Autodesk Inventor part; units mm, degrees
(part 2 of 3)
  spline S168 degree 2 poles (47.2484, 57.1416) (47.3031, 57.1416) (47.4113, 57.1684) (47.4635, 57.189) knots 0 0 0 1 2 2 2
  spline S169 degree 2 poles (47.4635, 57.189) (47.5122, 57.2097) (47.5839, 57.2534) (47.6118, 57.2729) knots 0 0 0 1 2 2 2
  line L293 (47.6118, 57.2729) -> (47.624, 57.2729)
  line L294 (47.624, 57.2729) -> (47.624, 57.0602)
  spline S170 degree 2 poles (47.624, 57.0602) (47.5583, 57.0249) (47.3335, 56.9678) (47.2326, 56.9678) knots 0 0 0 1 2 2 2
  spline S171 degree 2 poles (47.2326, 56.9678) (47.1305, 56.9678) (46.9785, 57.0091) (46.9165, 57.0529) knots 0 0 0 1 2 2 2
  spline S172 degree 2 poles (46.9165, 57.0529) (46.8509, 57.1003) (46.7828, 57.2376) (46.7828, 57.33) knots 0 0 0 1 2 2 2
  spline S173 degree 2 poles (46.7828, 57.33) (46.7828, 57.454) (46.9457, 57.6412) (47.06, 57.6655) knots 0 0 0 1 2 2 2
  line L295 (47.06, 57.6655) -> (47.06, 57.6801)
  spline S174 degree 2 poles (47.06, 57.6801) (47.0126, 57.6898) (46.9044, 57.7336) (46.8582, 57.7774) knots 0 0 0 1 2 2 2
  spline S175 degree 2 poles (46.8582, 57.7774) (46.812, 57.8199) (46.7536, 57.956) (46.7536, 58.0545) knots 0 0 0 1 2 2 2
  spline S176 degree 2 poles (46.7536, 58.0545) (46.7536, 58.1554) (46.8229, 58.3268) (46.8861, 58.3924) knots 0 0 0 1 2 2 2
  spline S177 degree 2 poles (46.8861, 58.3924) (46.9518, 58.4605) (47.1378, 58.531) (47.2557, 58.531) knots 0 0 0 1 2 2 2
  spline S178 degree 2 poles (47.2557, 58.531) (47.3687, 58.531) (47.59, 58.4763) (47.6653, 58.4386) knots 0 0 0 1 2 2 2
  line L296 (47.6653, 58.4386) -> (47.6653, 58.2259)
  line L297 (47.6653, 58.2259) -> (47.6507, 58.2259)
  spline S179 degree 2 poles (47.6507, 58.2259) (47.5875, 58.2721) (47.3736, 58.3572) (47.2678, 58.3572) knots 0 0 0 1 2 2 2
  spline S180 degree 2 poles (47.2678, 58.3572) (47.2058, 58.3572) (47.0818, 58.3183) (47.0405, 58.2733) knots 0 0 0 1 2 2 2
  spline S181 degree 2 poles (47.0405, 58.2733) (47.0004, 58.2283) (46.9579, 58.1214) (46.9579, 58.0399) knots 0 0 0 1 2 2 2
  spline S182 degree 2 poles (46.9579, 58.0399) (46.9579, 57.9585) (47.0053, 57.8527) (47.0478, 57.8223) knots 0 0 0 1 2 2 2
  spline S183 degree 2 poles (47.0478, 57.8223) (47.0904, 57.7919) (47.2058, 57.7688) (47.2739, 57.7688) knots 0 0 0 1 2 2 2
  line L298 (47.2739, 57.7688) -> (47.359, 57.7688)
  line L299 (47.359, 57.7688) -> (47.359, 57.6023)
  line L300 (47.359, 57.6023) -> (47.2921, 57.6023)
  spline S184 degree 2 poles (47.2921, 57.6023) (47.1572, 57.6023) (46.987, 57.4735) (46.987, 57.3507) knots 0 0 0 1 2 2 2
  spline S185 degree 2 poles (46.987, 57.3507) (46.987, 57.2936) (47.0308, 57.2121) (47.066, 57.1878) knots 0 0 0 1 2 2 2
  spline S186 degree 2 poles (47.066, 57.1878) (47.1037, 57.1623) (47.1961, 57.1416) (47.2484, 57.1416) knots 0 0 0 1 2 2 2
  line L301 (49.0097, 60.9994) -> (48.5041, 59.4994)
  line L302 (48.5041, 59.4994) -> (48.2585, 59.4994)
  line L303 (48.2585, 59.4994) -> (47.7528, 60.9994)
  line L304 (47.7528, 60.9994) -> (47.9631, 60.9994)
  line L305 (47.9631, 60.9994) -> (48.0993, 60.58)
  line L306 (48.0993, 60.58) -> (48.6718, 60.58)
  line L307 (48.6718, 60.58) -> (48.8079, 60.9994)
  line L308 (48.8079, 60.9994) -> (49.0097, 60.9994)
  line L309 (48.154, 60.4098) -> (48.3861, 59.7036)
  line L310 (48.3861, 59.7036) -> (48.6171, 60.4098)
  line L311 (48.6171, 60.4098) -> (48.154, 60.4098)
  line L312 (46.688, 60.484) -> (46.8667, 60.484)
  line L313 (46.8667, 60.484) -> (46.8667, 60.9994)
  line L314 (46.8667, 60.9994) -> (47.06, 60.9994)
  line L315 (47.06, 60.9994) -> (47.06, 60.484)
  line L316 (47.06, 60.484) -> (47.7224, 60.484)
  line L317 (47.7224, 60.484) -> (47.7224, 60.2725)
  line L318 (47.7224, 60.2725) -> (47.0515, 59.4994)
  line L319 (47.0515, 59.4994) -> (46.8667, 59.4994)
  line L320 (46.8667, 59.4994) -> (46.8667, 60.3223)
  line L321 (46.8667, 60.3223) -> (46.688, 60.3223)
  line L322 (46.688, 60.3223) -> (46.688, 60.484)
  line L323 (47.06, 60.3223) -> (47.06, 59.7364)
  line L324 (47.06, 59.7364) -> (47.5644, 60.3223)
  line L325 (47.5644, 60.3223) -> (47.06, 60.3223)
  line L326 (49.0097, 63.4994) -> (48.5041, 61.9994)
  line L327 (48.5041, 61.9994) -> (48.2585, 61.9994)
  line L328 (48.2585, 61.9994) -> (47.7528, 63.4994)
  line L329 (47.7528, 63.4994) -> (47.9631, 63.4994)
  line L330 (47.9631, 63.4994) -> (48.0993, 63.08)
  line L331 (48.0993, 63.08) -> (48.6718, 63.08)
  line L332 (48.6718, 63.08) -> (48.8079, 63.4994)
  line L333 (48.8079, 63.4994) -> (49.0097, 63.4994)
  line L334 (48.154, 62.9098) -> (48.3861, 62.2036)
  line L335 (48.3861, 62.2036) -> (48.6171, 62.9098)
  line L336 (48.6171, 62.9098) -> (48.154, 62.9098)
  spline S187 degree 2 poles (46.7439, 63.0229) (46.7439, 63.1311) (46.8132, 63.3158) (46.8764, 63.3839) knots 0 0 0 1 2 2 2
  spline S188 degree 2 poles (46.8764, 63.3839) (46.9396, 63.452) (47.128, 63.531) (47.2447, 63.531) knots 0 0 0 1 2 2 2
  spline S189 degree 2 poles (47.2447, 63.531) (47.3517, 63.531) (47.5608, 63.4836) (47.6374, 63.4459) knots 0 0 0 1 2 2 2
  line L337 (47.6374, 63.4459) -> (47.6374, 63.2332)
  line L338 (47.6374, 63.2332) -> (47.6228, 63.2332)
  spline S190 degree 2 poles (47.6228, 63.2332) (47.5997, 63.2502) (47.5134, 63.294) (47.4611, 63.3134) knots 0 0 0 1 2 2 2
  spline S191 degree 2 poles (47.4611, 63.3134) (47.4015, 63.3341) (47.3031, 63.3572) (47.2411, 63.3572) knots 0 0 0 1 2 2 2
  spline S192 degree 2 poles (47.2411, 63.3572) (47.1803, 63.3572) (47.066, 63.3134) (47.0247, 63.266) knots 0 0 0 1 2 2 2
  spline S193 degree 2 poles (47.0247, 63.266) (46.987, 63.221) (46.9481, 63.1019) (46.9481, 63.0217) knots 0 0 0 1 2 2 2
  spline S194 degree 2 poles (46.9481, 63.0217) (46.9481, 62.9415) (46.9919, 62.8393) (47.0332, 62.8053) knots 0 0 0 1 2 2 2
  spline S195 degree 2 poles (47.0332, 62.8053) (47.0758, 62.7676) (47.2022, 62.736) (47.2788, 62.736) knots 0 0 0 1 2 2 2
  spline S196 degree 2 poles (47.2788, 62.736) (47.3614, 62.736) (47.5255, 62.7615) (47.5754, 62.7725) knots 0 0 0 1 2 2 2
  line L339 (47.5754, 62.7725) -> (47.5754, 61.9994)
  line L340 (47.5754, 61.9994) -> (46.7524, 61.9994)
  line L341 (46.7524, 61.9994) -> (46.7524, 62.1756)
  line L342 (46.7524, 62.1756) -> (47.3821, 62.1756)
  line L343 (47.3821, 62.1756) -> (47.3821, 62.5756)
  spline S197 degree 2 poles (47.3821, 62.5756) (47.3456, 62.5707) (47.2751, 62.5671) (47.2459, 62.5671) knots 0 0 0 1 2 2 2
  spline S198 degree 2 poles (47.2459, 62.5671) (47.1305, 62.5671) (46.9712, 62.6047) (46.8983, 62.6607) knots 0 0 0 1 2 2 2
  spline S199 degree 2 poles (46.8983, 62.6607) (46.8241, 62.7166) (46.7439, 62.8868) (46.7439, 63.0229) knots 0 0 0 1 2 2 2
  line L344 (8.7601, 25.608) -> (8.2545, 24.108)
  line L345 (8.2545, 24.108) -> (8.0089, 24.108)
  line L346 (8.0089, 24.108) -> (7.5032, 25.608)
  line L347 (7.5032, 25.608) -> (7.7135, 25.608)
  line L348 (7.7135, 25.608) -> (7.8497, 25.1886)
  line L349 (7.8497, 25.1886) -> (8.4222, 25.1886)
  line L350 (8.4222, 25.1886) -> (8.5583, 25.608)
  line L351 (8.5583, 25.608) -> (8.7601, 25.608)
  line L352 (7.9044, 25.0184) -> (8.1365, 24.3122)
  line L353 (8.1365, 24.3122) -> (8.3675, 25.0184)
  line L354 (8.3675, 25.0184) -> (7.9044, 25.0184)
  line L355 (6.2002, 25.608) -> (6.4591, 25.608)
  line L356 (6.4591, 25.608) -> (6.9331, 25.0111)
  line L357 (6.9331, 25.0111) -> (7.1617, 25.0111)
  line L358 (7.1617, 25.0111) -> (7.1617, 25.608)
  line L359 (7.1617, 25.608) -> (7.361, 25.608)
  line L360 (7.361, 25.608) -> (7.361, 24.108)
  line L361 (7.361, 24.108) -> (6.9745, 24.108)
  spline S200 degree 2 poles (6.9745, 24.108) (6.8456, 24.108) (6.6718, 24.1359) (6.5928, 24.187) knots 0 0 0 1 2 2 2
  spline S201 degree 2 poles (6.5928, 24.187) (6.5138, 24.238) (6.4226, 24.3973) (6.4226, 24.5152) knots 0 0 0 1 2 2 2
  spline S202 degree 2 poles (6.4226, 24.5152) (6.4226, 24.6793) (6.5904, 24.9017) (6.7338, 24.9552) knots 0 0 0 1 2 2 2
  line L362 (6.7338, 24.9552) -> (6.2002, 25.608)
  spline S203 degree 2 poles (6.6305, 24.531) (6.6305, 24.4654) (6.6767, 24.3645) (6.7253, 24.3316) knots 0 0 0 1 2 2 2
  spline S204 degree 2 poles (6.7253, 24.3316) (6.7678, 24.3037) (6.8809, 24.2806) (6.9635, 24.2806) knots 0 0 0 1 2 2 2
  line L363 (6.9635, 24.2806) -> (7.1617, 24.2806)
  line L364 (7.1617, 24.2806) -> (7.1617, 24.8446)
  line L365 (7.1617, 24.8446) -> (6.9866, 24.8446)
  spline S205 degree 2 poles (6.9866, 24.8446) (6.9003, 24.8446) (6.763, 24.8142) (6.7156, 24.7668) knots 0 0 0 1 2 2 2
  spline S206 degree 2 poles (6.7156, 24.7668) (6.6718, 24.7255) (6.6305, 24.6088) (6.6305, 24.531) knots 0 0 0 1 2 2 2
  line L366 (6.081, 25.608) -> (6.081, 24.108)
  line L367 (6.081, 24.108) -> (5.1426, 24.108)
  line L368 (5.1426, 24.108) -> (5.1426, 24.2855)
  line L369 (5.1426, 24.2855) -> (5.8817, 24.2855)
  line L370 (5.8817, 24.2855) -> (5.8817, 24.6963)
  line L371 (5.8817, 24.6963) -> (5.1925, 24.6963)
  line L372 (5.1925, 24.6963) -> (5.1925, 24.8738)
  line L373 (5.1925, 24.8738) -> (5.8817, 24.8738)
  line L374 (5.8817, 24.8738) -> (5.8817, 25.4305)
  line L375 (5.8817, 25.4305) -> (5.1426, 25.4305)
  line L376 (5.1426, 25.4305) -> (5.1426, 25.608)
  line L377 (5.1426, 25.608) -> (6.081, 25.608)
  line L378 (4.0267, 24.2855) -> (4.7245, 24.2855)
  line L379 (4.7245, 24.2855) -> (4.7245, 24.7085)
  line L380 (4.7245, 24.7085) -> (4.0559, 24.7085)
  line L381 (4.0559, 24.7085) -> (4.0559, 24.8859)
  line L382 (4.0559, 24.8859) -> (4.7245, 24.8859)
  line L383 (4.7245, 24.8859) -> (4.7245, 25.608)
  line L384 (4.7245, 25.608) -> (4.9238, 25.608)
  line L385 (4.9238, 25.608) -> (4.9238, 24.108)
  line L386 (4.9238, 24.108) -> (4.0267, 24.108)
  line L387 (4.0267, 24.108) -> (4.0267, 24.2855)
  spline S207 degree 2 poles (7.3732, 28.1372) (7.5324, 28.1372) (7.7962, 28.0399) (7.891, 27.9415) knots 0 0 0 1 2 2 2
  spline S208 degree 2 poles (7.891, 27.9415) (7.9858, 27.8418) (8.0867, 27.5476) (8.0867, 27.3568) knots 0 0 0 1 2 2 2
  spline S209 degree 2 poles (8.0867, 27.3568) (8.0867, 27.1756) (7.9846, 26.8888) (7.8898, 26.7867) knots 0 0 0 1 2 2 2
  spline S210 degree 2 poles (7.8898, 26.7867) (7.7986, 26.6882) (7.5312, 26.5812) (7.372, 26.5812) knots 0 0 0 1 2 2 2
  spline S211 degree 2 poles (7.372, 26.5812) (7.2954, 26.5812) (7.1568, 26.6031) (7.0936, 26.6226) knots 0 0 0 1 2 2 2
  spline S212 degree 2 poles (7.0936, 26.6226) (7.0425, 26.6372) (6.9186, 26.6906) (6.8809, 26.7101) knots 0 0 0 1 2 2 2
  line L388 (6.8809, 26.7101) -> (6.8809, 26.9508)
  line L389 (6.8809, 26.9508) -> (6.8979, 26.9508)
  spline S213 degree 2 poles (6.8979, 26.9508) (6.9356, 26.9179) (7.0146, 26.8584) (7.0875, 26.8244) knots 0 0 0 1 2 2 2
  spline S214 degree 2 poles (7.0875, 26.8244) (7.1483, 26.794) (7.3051, 26.7538) (7.3951, 26.7538) knots 0 0 0 1 2 2 2
  spline S215 degree 2 poles (7.3951, 26.7538) (7.6114, 26.7538) (7.8788, 27.0796) (7.8788, 27.3507) knots 0 0 0 1 2 2 2
  spline S216 degree 2 poles (7.8788, 27.3507) (7.8788, 27.5014) (7.8083, 27.7275) (7.7415, 27.8053) knots 0 0 0 1 2 2 2
  spline S217 degree 2 poles (7.7415, 27.8053) (7.6771, 27.8831) (7.4947, 27.9645) (7.3805, 27.9645) knots 0 0 0 1 2 2 2
  spline S218 degree 2 poles (7.3805, 27.9645) (7.2966, 27.9645) (7.1288, 27.9402) (7.0717, 27.9159) knots 0 0 0 1 2 2 2
  line L390 (7.0717, 27.9159) -> (7.0717, 27.5282)
  line L391 (7.0717, 27.5282) -> (7.4194, 27.5282)
  line L392 (7.4194, 27.5282) -> (7.4194, 27.3531)
  line L393 (7.4194, 27.3531) -> (6.8748, 27.3531)
  line L394 (6.8748, 27.3531) -> (6.8748, 28.0083)
  spline S219 degree 2 poles (6.8748, 28.0083) (6.9125, 28.0253) (7.0413, 28.0776) (7.096, 28.0934) knots 0 0 0 1 2 2 2
  spline S220 degree 2 poles (7.096, 28.0934) (7.1702, 28.1153) (7.2893, 28.1372) (7.3732, 28.1372) knots 0 0 0 1 2 2 2
  line L395 (5.5511, 28.108) -> (5.7747, 28.108)
  line L396 (5.7747, 28.108) -> (6.4384, 26.8146)
  line L397 (6.4384, 26.8146) -> (6.4384, 28.108)
  line L398 (6.4384, 28.108) -> (6.6244, 28.108)
  line L399 (6.6244, 28.108) -> (6.6244, 26.608)
  line L400 (6.6244, 26.608) -> (6.3412, 26.608)
  line L401 (6.3412, 26.608) -> (5.737, 27.7956)
  line L402 (5.737, 27.7956) -> (5.737, 26.608)
  line L403 (5.737, 26.608) -> (5.5511, 26.608)
  line L404 (5.5511, 26.608) -> (5.5511, 28.108)
  spline S221 degree 2 poles (4.0644, 27.3592) (4.0644, 27.5646) (4.231, 27.8953) (4.3707, 27.9876) knots 0 0 0 1 2 2 2
  spline S222 degree 2 poles (4.3707, 27.9876) (4.485, 28.0594) (4.7196, 28.108) (4.9019, 28.108) knots 0 0 0 1 2 2 2
  line L405 (4.9019, 28.108) -> (5.2472, 28.108)
  line L406 (5.2472, 28.108) -> (5.2472, 26.608)
  line L407 (5.2472, 26.608) -> (4.9056, 26.608)
  spline S223 degree 2 poles (4.9056, 26.608) (4.6941, 26.608) (4.4534, 26.6712) (4.3683, 26.7271) knots 0 0 0 1 2 2 2
  spline S224 degree 2 poles (4.3683, 26.7271) (4.2237, 26.8231) (4.0644, 27.1404) (4.0644, 27.3592) knots 0 0 0 1 2 2 2
  spline S225 degree 2 poles (4.2723, 27.3568) (4.2723, 27.1842) (4.3865, 26.9398) (4.4996, 26.8705) knots 0 0 0 1 2 2 2
  spline S226 degree 2 poles (4.4996, 26.8705) (4.5798, 26.8231) (4.7609, 26.7806) (4.8959, 26.7806) knots 0 0 0 1 2 2 2
  line L408 (4.8959, 26.7806) -> (5.0478, 26.7806)
  line L409 (5.0478, 26.7806) -> (5.0478, 27.9354)
  line L410 (5.0478, 27.9354) -> (4.8959, 27.9354)
  spline S227 degree 2 poles (4.8959, 27.9354) (4.7634, 27.9354) (4.5628, 27.8928) (4.4814, 27.8357) knots 0 0 0 1 2 2 2
  spline S228 degree 2 poles (4.4814, 27.8357) (4.3768, 27.7652) (4.2723, 27.5318) (4.2723, 27.3568) knots 0 0 0 1 2 2 2
  line L411 (5.2921, 30.608) -> (6.0239, 30.608)
  line L412 (6.0239, 30.608) -> (6.0239, 30.4548)
  line L413 (6.0239, 30.4548) -> (5.7516, 30.4548)
  line L414 (5.7516, 30.4548) -> (5.7516, 29.4496)
  line L415 (5.7516, 29.4496) -> (6.0239, 29.4496)
  line L416 (6.0239, 29.4496) -> (6.0239, 29.3122)
  spline S229 degree 2 poles (6.0239, 29.3122) (5.8695, 29.3122) (5.7237, 29.2247) (5.7139, 29.1031) knots 0 0 0 1 2 2 2
  line L417 (5.7139, 29.1031) -> (5.5583, 29.1031)
  line L418 (5.5583, 29.1031) -> (5.5583, 30.4548)
  line L419 (5.5583, 30.4548) -> (5.2921, 30.4548)
  line L420 (5.2921, 30.4548) -> (5.2921, 30.608)
  spline S230 degree 2 poles (4.6114, 29.2502) (4.6661, 29.2502) (4.7743, 29.2769) (4.8266, 29.2976) knots 0 0 0 1 2 2 2
  spline S231 degree 2 poles (4.8266, 29.2976) (4.8752, 29.3183) (4.9469, 29.362) (4.9749, 29.3815) knots 0 0 0 1 2 2 2
  line L421 (4.9749, 29.3815) -> (4.987, 29.3815)
  line L422 (4.987, 29.3815) -> (4.987, 29.1688)
  spline S232 degree 2 poles (4.987, 29.1688) (4.9214, 29.1335) (4.6965, 29.0764) (4.5956, 29.0764) knots 0 0 0 1 2 2 2
  spline S233 degree 2 poles (4.5956, 29.0764) (4.4935, 29.0764) (4.3416, 29.1177) (4.2796, 29.1615) knots 0 0 0 1 2 2 2
  spline S234 degree 2 poles (4.2796, 29.1615) (4.2139, 29.2089) (4.1459, 29.3462) (4.1459, 29.4386) knots 0 0 0 1 2 2 2
  spline S235 degree 2 poles (4.1459, 29.4386) (4.1459, 29.5626) (4.3088, 29.7498) (4.423, 29.7741) knots 0 0 0 1 2 2 2
  line L423 (4.423, 29.7741) -> (4.423, 29.7887)
  spline S236 degree 2 poles (4.423, 29.7887) (4.3756, 29.7984) (4.2674, 29.8422) (4.2212, 29.8859) knots 0 0 0 1 2 2 2
  spline S237 degree 2 poles (4.2212, 29.8859) (4.175, 29.9285) (4.1167, 30.0646) (4.1167, 30.1631) knots 0 0 0 1 2 2 2
  spline S238 degree 2 poles (4.1167, 30.1631) (4.1167, 30.264) (4.186, 30.4354) (4.2492, 30.501) knots 0 0 0 1 2 2 2
  spline S239 degree 2 poles (4.2492, 30.501) (4.3148, 30.5691) (4.5008, 30.6396) (4.6187, 30.6396) knots 0 0 0 1 2 2 2
  spline S240 degree 2 poles (4.6187, 30.6396) (4.7318, 30.6396) (4.953, 30.5849) (5.0284, 30.5472) knots 0 0 0 1 2 2 2
  line L424 (5.0284, 30.5472) -> (5.0284, 30.3345)
  line L425 (5.0284, 30.3345) -> (5.0138, 30.3345)
  spline S241 degree 2 poles (5.0138, 30.3345) (4.9506, 30.3807) (4.7366, 30.4658) (4.6309, 30.4658) knots 0 0 0 1 2 2 2
  spline S242 degree 2 poles (4.6309, 30.4658) (4.5689, 30.4658) (4.4449, 30.4269) (4.4036, 30.3819) knots 0 0 0 1 2 2 2
  spline S243 degree 2 poles (4.4036, 30.3819) (4.3635, 30.3369) (4.3209, 30.2299) (4.3209, 30.1485) knots 0 0 0 1 2 2 2
  spline S244 degree 2 poles (4.3209, 30.1485) (4.3209, 30.0671) (4.3683, 29.9613) (4.4109, 29.9309) knots 0 0 0 1 2 2 2
  spline S245 degree 2 poles (4.4109, 29.9309) (4.4534, 29.9005) (4.5689, 29.8774) (4.637, 29.8774) knots 0 0 0 1 2 2 2
  line L426 (4.637, 29.8774) -> (4.722, 29.8774)
  line L427 (4.722, 29.8774) -> (4.722, 29.7109)
  line L428 (4.722, 29.7109) -> (4.6552, 29.7109)
  spline S246 degree 2 poles (4.6552, 29.7109) (4.5203, 29.7109) (4.3501, 29.5821) (4.3501, 29.4593) knots 0 0 0 1 2 2 2
  spline S247 degree 2 poles (4.3501, 29.4593) (4.3501, 29.4021) (4.3938, 29.3207) (4.4291, 29.2964) knots 0 0 0 1 2 2 2
  spline S248 degree 2 poles (4.4291, 29.2964) (4.4668, 29.2709) (4.5592, 29.2502) (4.6114, 29.2502) knots 0 0 0 1 2 2 2
  line L429 (5.2921, 33.108) -> (6.0239, 33.108)
  line L430 (6.0239, 33.108) -> (6.0239, 32.9548)
  line L431 (6.0239, 32.9548) -> (5.7516, 32.9548)
  line L432 (5.7516, 32.9548) -> (5.7516, 31.9496)
  line L433 (5.7516, 31.9496) -> (6.0239, 31.9496)
  line L434 (6.0239, 31.9496) -> (6.0239, 31.8122)
  spline S249 degree 2 poles (6.0239, 31.8122) (5.8695, 31.8122) (5.7237, 31.7247) (5.7139, 31.6031) knots 0 0 0 1 2 2 2
  line L435 (5.7139, 31.6031) -> (5.5583, 31.6031)
  line L436 (5.5583, 31.6031) -> (5.5583, 32.9548)
  line L437 (5.5583, 32.9548) -> (5.2921, 32.9548)
  line L438 (5.2921, 32.9548) -> (5.2921, 33.108)
  line L439 (4.0912, 33.108) -> (5.0162, 33.108)
  line L440 (5.0162, 33.108) -> (5.0162, 32.8953)
  spline S250 degree 2 poles (5.0162, 32.8953) (4.9165, 32.8017) (4.7391, 32.6278) (4.654, 32.5342) knots 0 0 0 1 2 2 2
  spline S251 degree 2 poles (4.654, 32.5342) (4.4826, 32.3458) (4.3574, 32.1197) (4.3574, 31.9994) knots 0 0 0 1 2 2 2
  spline S252 degree 2 poles (4.3574, 31.9994) (4.3574, 31.9362) (4.3963, 31.8414) (4.4315, 31.811) knots 0 0 0 1 2 2 2
  spline S253 degree 2 poles (4.4315, 31.811) (4.4668, 31.7806) (4.5592, 31.7502) (4.6151, 31.7502) knots 0 0 0 1 2 2 2
  spline S254 degree 2 poles (4.6151, 31.7502) (4.6686, 31.7502) (4.778, 31.7769) (4.8278, 31.7976) knots 0 0 0 1 2 2 2
  spline S255 degree 2 poles (4.8278, 31.7976) (4.8703, 31.8146) (4.9494, 31.8632) (4.9737, 31.8803) knots 0 0 0 1 2 2 2
  line L441 (4.9737, 31.8803) -> (4.9846, 31.8803)
  line L442 (4.9846, 31.8803) -> (4.9846, 31.6663)
  spline S256 degree 2 poles (4.9846, 31.6663) (4.9226, 31.6359) (4.7002, 31.5764) (4.6005, 31.5764) knots 0 0 0 1 2 2 2
  spline S257 degree 2 poles (4.6005, 31.5764) (4.3902, 31.5764) (4.1532, 31.7988) (4.1532, 31.9885) knots 0 0 0 1 2 2 2
  spline S258 degree 2 poles (4.1532, 31.9885) (4.1532, 32.0772) (4.1945, 32.2255) (4.231, 32.2887) knots 0 0 0 1 2 2 2
  spline S259 degree 2 poles (4.231, 32.2887) (4.2674, 32.3543) (4.3732, 32.4832) (4.4315, 32.5452) knots 0 0 0 1 2 2 2
  spline S260 degree 2 poles (4.4315, 32.5452) (4.5263, 32.6485) (4.7585, 32.8697) (4.8278, 32.9342) knots 0 0 0 1 2 2 2
  line L443 (4.8278, 32.9342) -> (4.0912, 32.9342)
  line L444 (4.0912, 32.9342) -> (4.0912, 33.108)
  spline S261 degree 2 poles (6.3861, 34.6756) (6.3886, 34.7778) (6.4263, 34.9686) (6.4676, 35.044) knots 0 0 0 1 2 2 2
  spline S262 degree 2 poles (6.4676, 35.044) (6.5089, 35.1169) (6.6317, 35.2093) (6.7301, 35.2093) knots 0 0 0 1 2 2 2
  spline S263 degree 2 poles (6.7301, 35.2093) (6.7885, 35.2093) (6.8797, 35.1777) (6.9149, 35.1534) knots 0 0 0 1 2 2 2
  spline S264 degree 2 poles (6.9149, 35.1534) (6.9502, 35.1278) (7.0146, 35.0573) (7.0401, 35.0269) knots 0 0 0 1 2 2 2
  spline S265 degree 2 poles (7.0401, 35.0269) (7.0669, 34.9941) (7.1191, 34.9248) (7.1447, 34.8993) knots 0 0 0 1 2 2 2
  spline S266 degree 2 poles (7.1447, 34.8993) (7.1726, 34.8714) (7.231, 34.8373) (7.2674, 34.8373) knots 0 0 0 1 2 2 2
  spline S267 degree 2 poles (7.2674, 34.8373) (7.3185, 34.8373) (7.3853, 34.8908) (7.4072, 34.9431) knots 0 0 0 1 2 2 2
  spline S268 degree 2 poles (7.4072, 34.9431) (7.4279, 34.9929) (7.4461, 35.1327) (7.4485, 35.2093) knots 0 0 0 1 2 2 2
  line L445 (7.4485, 35.2093) -> (7.6175, 35.2093)
  spline S269 degree 2 poles (7.6175, 35.2093) (7.6151, 35.1047) (7.5762, 34.9139) (7.5373, 34.841) knots 0 0 0 1 2 2 2
  spline S270 degree 2 poles (7.5373, 34.841) (7.4972, 34.7656) (7.3635, 34.6756) (7.2723, 34.6756) knots 0 0 0 1 2 2 2
  spline S271 degree 2 poles (7.2723, 34.6756) (7.2127, 34.6756) (7.1203, 34.7073) (7.0851, 34.7328) knots 0 0 0 1 2 2 2
  spline S272 degree 2 poles (7.0851, 34.7328) (7.0498, 34.7583) (6.9903, 34.8227) (6.9623, 34.858) knots 0 0 0 1 2 2 2
  spline S273 degree 2 poles (6.9623, 34.858) (6.9404, 34.8847) (6.8784, 34.9637) (6.8578, 34.9856) knots 0 0 0 1 2 2 2
  spline S274 degree 2 poles (6.8578, 34.9856) (6.8286, 35.016) (6.769, 35.0476) (6.7362, 35.0476) knots 0 0 0 1 2 2 2
  spline S275 degree 2 poles (6.7362, 35.0476) (6.6852, 35.0476) (6.6159, 34.9917) (6.5964, 34.9431) knots 0 0 0 1 2 2 2
  spline S276 degree 2 poles (6.5964, 34.9431) (6.5758, 34.8932) (6.5575, 34.7583) (6.5551, 34.6756) knots 0 0 0 1 2 2 2
  line L446 (6.5551, 34.6756) -> (6.3861, 34.6756)
  line L447 (5.2921, 35.608) -> (6.0239, 35.608)
  line L448 (6.0239, 35.608) -> (6.0239, 35.4548)
  line L449 (6.0239, 35.4548) -> (5.7516, 35.4548)
  line L450 (5.7516, 35.4548) -> (5.7516, 34.4496)
  line L451 (5.7516, 34.4496) -> (6.0239, 34.4496)
  line L452 (6.0239, 34.4496) -> (6.0239, 34.3122)
  spline S277 degree 2 poles (6.0239, 34.3122) (5.8695, 34.3122) (5.7237, 34.2247) (5.7139, 34.1031) knots 0 0 0 1 2 2 2
  line L453 (5.7139, 34.1031) -> (5.5583, 34.1031)
  line L454 (5.5583, 34.1031) -> (5.5583, 35.4548)
  line L455 (5.5583, 35.4548) -> (5.2921, 35.4548)
  line L456 (5.2921, 35.4548) -> (5.2921, 35.608)
  line L457 (4.1665, 35.608) -> (4.8983, 35.608)
  line L458 (4.8983, 35.608) -> (4.8983, 35.4548)
  line L459 (4.8983, 35.4548) -> (4.626, 35.4548)
  line L460 (4.626, 35.4548) -> (4.626, 34.4496)
  line L461 (4.626, 34.4496) -> (4.8983, 34.4496)
  line L462 (4.8983, 34.4496) -> (4.8983, 34.3122)
  spline S278 degree 2 poles (4.8983, 34.3122) (4.7439, 34.3122) (4.5981, 34.2247) (4.5883, 34.1031) knots 0 0 0 1 2 2 2
  line L463 (4.5883, 34.1031) -> (4.4327, 34.1031)
  line L464 (4.4327, 34.1031) -> (4.4327, 35.4548)
  line L465 (4.4327, 35.4548) -> (4.1665, 35.4548)
  line L466 (4.1665, 35.4548) -> (4.1665, 35.608)
  spline S279 degree 2 poles (6.3861, 37.1756) (6.3886, 37.2778) (6.4263, 37.4686) (6.4676, 37.544) knots 0 0 0 1 2 2 2
  spline S280 degree 2 poles (6.4676, 37.544) (6.5089, 37.6169) (6.6317, 37.7093) (6.7301, 37.7093) knots 0 0 0 1 2 2 2
  spline S281 degree 2 poles (6.7301, 37.7093) (6.7885, 37.7093) (6.8797, 37.6777) (6.9149, 37.6534) knots 0 0 0 1 2 2 2
  spline S282 degree 2 poles (6.9149, 37.6534) (6.9502, 37.6278) (7.0146, 37.5573) (7.0401, 37.5269) knots 0 0 0 1 2 2 2
  spline S283 degree 2 poles (7.0401, 37.5269) (7.0669, 37.4941) (7.1191, 37.4248) (7.1447, 37.3993) knots 0 0 0 1 2 2 2
  spline S284 degree 2 poles (7.1447, 37.3993) (7.1726, 37.3714) (7.231, 37.3373) (7.2674, 37.3373) knots 0 0 0 1 2 2 2
  spline S285 degree 2 poles (7.2674, 37.3373) (7.3185, 37.3373) (7.3853, 37.3908) (7.4072, 37.4431) knots 0 0 0 1 2 2 2
  spline S286 degree 2 poles (7.4072, 37.4431) (7.4279, 37.4929) (7.4461, 37.6327) (7.4485, 37.7093) knots 0 0 0 1 2 2 2
  line L467 (7.4485, 37.7093) -> (7.6175, 37.7093)
  spline S287 degree 2 poles (7.6175, 37.7093) (7.6151, 37.6047) (7.5762, 37.4139) (7.5373, 37.341) knots 0 0 0 1 2 2 2
  spline S288 degree 2 poles (7.5373, 37.341) (7.4972, 37.2656) (7.3635, 37.1756) (7.2723, 37.1756) knots 0 0 0 1 2 2 2
  spline S289 degree 2 poles (7.2723, 37.1756) (7.2127, 37.1756) (7.1203, 37.2073) (7.0851, 37.2328) knots 0 0 0 1 2 2 2
  spline S290 degree 2 poles (7.0851, 37.2328) (7.0498, 37.2583) (6.9903, 37.3227) (6.9623, 37.358) knots 0 0 0 1 2 2 2
  spline S291 degree 2 poles (6.9623, 37.358) (6.9404, 37.3847) (6.8784, 37.4637) (6.8578, 37.4856) knots 0 0 0 1 2 2 2
  spline S292 degree 2 poles (6.8578, 37.4856) (6.8286, 37.516) (6.769, 37.5476) (6.7362, 37.5476) knots 0 0 0 1 2 2 2
  spline S293 degree 2 poles (6.7362, 37.5476) (6.6852, 37.5476) (6.6159, 37.4917) (6.5964, 37.4431) knots 0 0 0 1 2 2 2
  spline S294 degree 2 poles (6.5964, 37.4431) (6.5758, 37.3932) (6.5575, 37.2583) (6.5551, 37.1756) knots 0 0 0 1 2 2 2
  line L468 (6.5551, 37.1756) -> (6.3861, 37.1756)
  line L469 (5.2921, 38.108) -> (6.0239, 38.108)
  line L470 (6.0239, 38.108) -> (6.0239, 37.9548)
  line L471 (6.0239, 37.9548) -> (5.7516, 37.9548)
  line L472 (5.7516, 37.9548) -> (5.7516, 36.9496)
  line L473 (5.7516, 36.9496) -> (6.0239, 36.9496)
  line L474 (6.0239, 36.9496) -> (6.0239, 36.8122)
  spline S295 degree 2 poles (6.0239, 36.8122) (5.8695, 36.8122) (5.7237, 36.7247) (5.7139, 36.6031) knots 0 0 0 1 2 2 2
  line L475 (5.7139, 36.6031) -> (5.5583, 36.6031)
  line L476 (5.5583, 36.6031) -> (5.5583, 37.9548)
  line L477 (5.5583, 37.9548) -> (5.2921, 37.9548)
  line L478 (5.2921, 37.9548) -> (5.2921, 38.108)
  spline S296 degree 2 poles (4.0827, 37.358) (4.0827, 37.7615) (4.3173, 38.1396) (4.5616, 38.1396) knots 0 0 0 1 2 2 2
  spline S297 degree 2 poles (4.5616, 38.1396) (4.8096, 38.1396) (5.0417, 37.7543) (5.0417, 37.3592) knots 0 0 0 1 2 2 2
  spline S298 degree 2 poles (5.0417, 37.3592) (5.0417, 36.9532) (4.8071, 36.5776) (4.5616, 36.5776) knots 0 0 0 1 2 2 2
  spline S299 degree 2 poles (4.5616, 36.5776) (4.3148, 36.5776) (4.0827, 36.9666) (4.0827, 37.358) knots 0 0 0 1 2 2 2
  spline S300 degree 2 poles (4.3404, 37.815) (4.3112, 37.7409) (4.2869, 37.5124) (4.2869, 37.358) knots 0 0 0 1 2 2 2
  spline S301 degree 2 poles (4.2869, 37.358) (4.2869, 37.2036) (4.3112, 36.9763) (4.3416, 36.8997) knots 0 0 0 1 2 2 2
  spline S302 degree 2 poles (4.3416, 36.8997) (4.372, 36.8231) (4.4777, 36.7441) (4.5616, 36.7441) knots 0 0 0 1 2 2 2
  spline S303 degree 2 poles (4.5616, 36.7441) (4.6455, 36.7441) (4.7536, 36.8231) (4.7853, 36.9021) knots 0 0 0 1 2 2 2
  spline S304 degree 2 poles (4.7853, 36.9021) (4.8156, 36.9787) (4.8375, 37.2121) (4.8375, 37.3592) knots 0 0 0 1 2 2 2
  spline S305 degree 2 poles (4.8375, 37.3592) (4.8375, 37.5172) (4.8181, 37.7287) (4.7865, 37.8114) knots 0 0 0 1 2 2 2
  spline S306 degree 2 poles (4.7865, 37.8114) (4.7573, 37.8892) (4.6491, 37.9731) (4.5616, 37.9731) knots 0 0 0 1 2 2 2
  spline S307 degree 2 poles (4.5616, 37.9731) (4.4789, 37.9731) (4.3707, 37.894) (4.3404, 37.815) knots 0 0 0 1 2 2 2
  spline S308 degree 2 poles (5.2605, 39.6756) (5.263, 39.7778) (5.3006, 39.9686) (5.342, 40.044) knots 0 0 0 1 2 2 2
  spline S309 degree 2 poles (5.342, 40.044) (5.3833, 40.1169) (5.5061, 40.2093) (5.6045, 40.2093) knots 0 0 0 1 2 2 2
  spline S310 degree 2 poles (5.6045, 40.2093) (5.6629, 40.2093) (5.7541, 40.1777) (5.7893, 40.1534) knots 0 0 0 1 2 2 2
  spline S311 degree 2 poles (5.7893, 40.1534) (5.8246, 40.1278) (5.889, 40.0573) (5.9145, 40.0269) knots 0 0 0 1 2 2 2
  spline S312 degree 2 poles (5.9145, 40.0269) (5.9412, 39.9941) (5.9935, 39.9248) (6.019, 39.8993) knots 0 0 0 1 2 2 2
  spline S313 degree 2 poles (6.019, 39.8993) (6.047, 39.8714) (6.1053, 39.8373) (6.1418, 39.8373) knots 0 0 0 1 2 2 2
  spline S314 degree 2 poles (6.1418, 39.8373) (6.1929, 39.8373) (6.2597, 39.8908) (6.2816, 39.9431) knots 0 0 0 1 2 2 2
  spline S315 degree 2 poles (6.2816, 39.9431) (6.3023, 39.9929) (6.3205, 40.1327) (6.3229, 40.2093) knots 0 0 0 1 2 2 2
  line L479 (6.3229, 40.2093) -> (6.4919, 40.2093)
  spline S316 degree 2 poles (6.4919, 40.2093) (6.4895, 40.1047) (6.4506, 39.9139) (6.4117, 39.841) knots 0 0 0 1 2 2 2
  spline S317 degree 2 poles (6.4117, 39.841) (6.3716, 39.7656) (6.2378, 39.6756) (6.1467, 39.6756) knots 0 0 0 1 2 2 2
  spline S318 degree 2 poles (6.1467, 39.6756) (6.0871, 39.6756) (5.9947, 39.7073) (5.9595, 39.7328) knots 0 0 0 1 2 2 2
  spline S319 degree 2 poles (5.9595, 39.7328) (5.9242, 39.7583) (5.8647, 39.8227) (5.8367, 39.858) knots 0 0 0 1 2 2 2
  spline S320 degree 2 poles (5.8367, 39.858) (5.8148, 39.8847) (5.7528, 39.9637) (5.7322, 39.9856) knots 0 0 0 1 2 2 2
  spline S321 degree 2 poles (5.7322, 39.9856) (5.703, 40.016) (5.6434, 40.0476) (5.6106, 40.0476) knots 0 0 0 1 2 2 2
  spline S322 degree 2 poles (5.6106, 40.0476) (5.5596, 40.0476) (5.4903, 39.9917) (5.4708, 39.9431) knots 0 0 0 1 2 2 2
  spline S323 degree 2 poles (5.4708, 39.9431) (5.4502, 39.8932) (5.4319, 39.7583) (5.4295, 39.6756) knots 0 0 0 1 2 2 2
  line L480 (5.4295, 39.6756) -> (5.2605, 39.6756)
  spline S324 degree 2 poles (5.0575, 39.5954) (5.0575, 39.4799) (4.9822, 39.2879) (4.9165, 39.2186) knots 0 0 0 1 2 2 2
  spline S325 degree 2 poles (4.9165, 39.2186) (4.8545, 39.1517) (4.6734, 39.0776) (4.581, 39.0776) knots 0 0 0 1 2 2 2
  spline S326 degree 2 poles (4.581, 39.0776) (4.4777, 39.0776) (4.31, 39.1469) (4.248, 39.2125) knots 0 0 0 1 2 2 2
  spline S327 degree 2 poles (4.248, 39.2125) (4.1702, 39.2952) (4.0851, 39.5626) (4.0851, 39.768) knots 0 0 0 1 2 2 2
  spline S328 degree 2 poles (4.0851, 39.768) (4.0851, 39.954) (4.169, 40.2871) (4.2504, 40.3977) knots 0 0 0 1 2 2 2
  spline S329 degree 2 poles (4.2504, 40.3977) (4.3367, 40.5144) (4.5798, 40.6372) (4.7573, 40.6372) knots 0 0 0 1 2 2 2
  spline S330 degree 2 poles (4.7573, 40.6372) (4.7974, 40.6372) (4.8886, 40.6286) (4.9275, 40.6165) knots 0 0 0 1 2 2 2
  line L481 (4.9275, 40.6165) -> (4.9275, 40.4232)
  line L482 (4.9275, 40.4232) -> (4.9177, 40.4232)
  spline S331 degree 2 poles (4.9177, 40.4232) (4.8922, 40.4378) (4.7853, 40.4633) (4.7306, 40.4633) knots 0 0 0 1 2 2 2
  spline S332 degree 2 poles (4.7306, 40.4633) (4.5336, 40.4633) (4.3088, 40.2032) (4.2929, 39.9625) knots 0 0 0 1 2 2 2
  spline S333 degree 2 poles (4.2929, 39.9625) (4.3732, 40.0172) (4.519, 40.0671) (4.6053, 40.0671) knots 0 0 0 1 2 2 2
  spline S334 degree 2 poles (4.6053, 40.0671) (4.688, 40.0671) (4.8254, 40.0306) (4.8947, 39.9783) knots 0 0 0 1 2 2 2
  spline S335 degree 2 poles (4.8947, 39.9783) (4.9749, 39.9163) (5.0575, 39.7279) (5.0575, 39.5954) knots 0 0 0 1 2 2 2
  spline S336 degree 2 poles (4.2881, 39.7231) (4.2881, 39.5711) (4.344, 39.3791) (4.3938, 39.3268) knots 0 0 0 1 2 2 2
  spline S337 degree 2 poles (4.3938, 39.3268) (4.4376, 39.2782) (4.5288, 39.2417) (4.5823, 39.2417) knots 0 0 0 1 2 2 2
  spline S338 degree 2 poles (4.5823, 39.2417) (4.7062, 39.2417) (4.8533, 39.4192) (4.8533, 39.5869) knots 0 0 0 1 2 2 2
  spline S339 degree 2 poles (4.8533, 39.5869) (4.8533, 39.6817) (4.8047, 39.8045) (4.7512, 39.8483) knots 0 0 0 1 2 2 2
  spline S340 degree 2 poles (4.7512, 39.8483) (4.7123, 39.8799) (4.6163, 39.9005) (4.5604, 39.9005) knots 0 0 0 1 2 2 2
  spline S341 degree 2 poles (4.5604, 39.9005) (4.4959, 39.9005) (4.3476, 39.8556) (4.2917, 39.8179) knots 0 0 0 1 2 2 2
  spline S342 degree 2 poles (4.2917, 39.8179) (4.2905, 39.8033) (4.2881, 39.7534) (4.2881, 39.7231) knots 0 0 0 1 2 2 2
  spline S343 degree 2 poles (4.5628, 43.142) (4.6746, 43.142) (4.8582, 43.0752) (4.9226, 43.0132) knots 0 0 0 1 2 2 2
  spline S344 degree 2 poles (4.9226, 43.0132) (4.9858, 42.9524) (5.0515, 42.7871) (5.0515, 42.6935) knots 0 0 0 1 2 2 2
  spline S345 degree 2 poles (5.0515, 42.6935) (5.0515, 42.5719) (4.9214, 42.3677) (4.7974, 42.3069) knots 0 0 0 1 2 2 2
  line L483 (4.7974, 42.3069) -> (4.7974, 42.3009)
  spline S346 degree 2 poles (4.7974, 42.3009) (4.908, 42.2364) (5.015, 42.0833) (5.015, 41.969) knots 0 0 0 1 2 2 2
  spline S347 degree 2 poles (5.015, 41.969) (5.015, 41.8) (4.7597, 41.5739) (4.5628, 41.5739) knots 0 0 0 1 2 2 2
  spline S348 degree 2 poles (4.5628, 41.5739) (4.3586, 41.5739) (4.1118, 41.7879) (4.1118, 41.9556) knots 0 0 0 1 2 2 2
  spline S349 degree 2 poles (4.1118, 41.9556) (4.1118, 42.0565) (4.2297, 42.2534) (4.3404, 42.3094) knots 0 0 0 1 2 2 2
  line L484 (4.3404, 42.3094) -> (4.3404, 42.3154)
  spline S350 degree 2 poles (4.3404, 42.3154) (4.2091, 42.3762) (4.0741, 42.5513) (4.0741, 42.6898) knots 0 0 0 1 2 2 2
  spline S351 degree 2 poles (4.0741, 42.6898) (4.0741, 42.8819) (4.3537, 43.142) (4.5628, 43.142) knots 0 0 0 1 2 2 2
  spline S352 degree 2 poles (4.2808, 42.7093) (4.2808, 42.6169) (4.3537, 42.5075) (4.4571, 42.4516) knots 0 0 0 1 2 2 2
  spline S353 degree 2 poles (4.4571, 42.4516) (4.4911, 42.4321) (4.6053, 42.3872) (4.6771, 42.358) knots 0 0 0 1 2 2 2
  spline S354 degree 2 poles (4.6771, 42.358) (4.7597, 42.4127) (4.8485, 42.5756) (4.8485, 42.6789) knots 0 0 0 1 2 2 2
  spline S355 degree 2 poles (4.8485, 42.6789) (4.8485, 42.815) (4.6844, 42.9925) (4.5604, 42.9925) knots 0 0 0 1 2 2 2
  spline S356 degree 2 poles (4.5604, 42.9925) (4.434, 42.9925) (4.2808, 42.8406) (4.2808, 42.7093) knots 0 0 0 1 2 2 2
  spline S357 degree 2 poles (4.3088, 41.9581) (4.3088, 41.8572) (4.4437, 41.7222) (4.564, 41.7222) knots 0 0 0 1 2 2 2
  spline S358 degree 2 poles (4.564, 41.7222) (4.6734, 41.7222) (4.8132, 41.8426) (4.8132, 41.9459) knots 0 0 0 1 2 2 2
  spline S359 degree 2 poles (4.8132, 41.9459) (4.8132, 42.0201) (4.7415, 42.1234) (4.6698, 42.1647) knots 0 0 0 1 2 2 2
  spline S360 degree 2 poles (4.6698, 42.1647) (4.6394, 42.1817) (4.5105, 42.2413) (4.4583, 42.2583) knots 0 0 0 1 2 2 2
  spline S361 degree 2 poles (4.4583, 42.2583) (4.3707, 42.1915) (4.3088, 42.0492) (4.3088, 41.9581) knots 0 0 0 1 2 2 2
  line L485 (4.0741, 44.7249) -> (4.7233, 46)
  line L486 (4.7233, 46) -> (4.9372, 46)
  line L487 (4.9372, 46) -> (4.2516, 44.6763)
  line L488 (4.2516, 44.6763) -> (5.0259, 44.6763)
  line L489 (5.0259, 44.6763) -> (5.0259, 44.5)
  line L490 (5.0259, 44.5) -> (4.0741, 44.5)
  line L491 (4.0741, 44.5) -> (4.0741, 44.7249)
  spline S362 degree 2 poles (5.2605, 47.5677) (5.263, 47.6698) (5.3006, 47.8606) (5.342, 47.936) knots 0 0 0 1 2 2 2
  spline S363 degree 2 poles (5.342, 47.936) (5.3833, 48.0089) (5.5061, 48.1013) (5.6045, 48.1013) knots 0 0 0 1 2 2 2
  spline S364 degree 2 poles (5.6045, 48.1013) (5.6629, 48.1013) (5.7541, 48.0697) (5.7893, 48.0454) knots 0 0 0 1 2 2 2
  spline S365 degree 2 poles (5.7893, 48.0454) (5.8246, 48.0199) (5.889, 47.9494) (5.9145, 47.919) knots 0 0 0 1 2 2 2
  spline S366 degree 2 poles (5.9145, 47.919) (5.9412, 47.8861) (5.9935, 47.8169) (6.019, 47.7913) knots 0 0 0 1 2 2 2
  spline S367 degree 2 poles (6.019, 47.7913) (6.047, 47.7634) (6.1053, 47.7293) (6.1418, 47.7293) knots 0 0 0 1 2 2 2
  spline S368 degree 2 poles (6.1418, 47.7293) (6.1929, 47.7293) (6.2597, 47.7828) (6.2816, 47.8351) knots 0 0 0 1 2 2 2
  spline S369 degree 2 poles (6.2816, 47.8351) (6.3023, 47.8849) (6.3205, 48.0247) (6.3229, 48.1013) knots 0 0 0 1 2 2 2
  line L492 (6.3229, 48.1013) -> (6.4919, 48.1013)
  spline S370 degree 2 poles (6.4919, 48.1013) (6.4895, 47.9968) (6.4506, 47.8059) (6.4117, 47.733) knots 0 0 0 1 2 2 2
  spline S371 degree 2 poles (6.4117, 47.733) (6.3716, 47.6576) (6.2378, 47.5677) (6.1467, 47.5677) knots 0 0 0 1 2 2 2
  spline S372 degree 2 poles (6.1467, 47.5677) (6.0871, 47.5677) (5.9947, 47.5993) (5.9595, 47.6248) knots 0 0 0 1 2 2 2
  spline S373 degree 2 poles (5.9595, 47.6248) (5.9242, 47.6503) (5.8647, 47.7147) (5.8367, 47.75) knots 0 0 0 1 2 2 2
  spline S374 degree 2 poles (5.8367, 47.75) (5.8148, 47.7767) (5.7528, 47.8558) (5.7322, 47.8776) knots 0 0 0 1 2 2 2
  spline S375 degree 2 poles (5.7322, 47.8776) (5.703, 47.908) (5.6434, 47.9396) (5.6106, 47.9396) knots 0 0 0 1 2 2 2
  spline S376 degree 2 poles (5.6106, 47.9396) (5.5596, 47.9396) (5.4903, 47.8837) (5.4708, 47.8351) knots 0 0 0 1 2 2 2
  spline S377 degree 2 poles (5.4708, 47.8351) (5.4502, 47.7853) (5.4319, 47.6503) (5.4295, 47.5677) knots 0 0 0 1 2 2 2
  line L493 (5.4295, 47.5677) -> (5.2605, 47.5677)
  spline S378 degree 2 poles (4.0681, 48.0138) (4.0681, 48.1293) (4.1447, 48.325) (4.2091, 48.3906) knots 0 0 0 1 2 2 2
  spline S379 degree 2 poles (4.2091, 48.3906) (4.2759, 48.4599) (4.4437, 48.5316) (4.5446, 48.5316) knots 0 0 0 1 2 2 2
  spline S380 degree 2 poles (4.5446, 48.5316) (4.6455, 48.5316) (4.812, 48.4635) (4.8752, 48.3955) knots 0 0 0 1 2 2 2
  spline S381 degree 2 poles (4.8752, 48.3955) (4.953, 48.314) (5.0405, 48.0405) (5.0405, 47.8412) knots 0 0 0 1 2 2 2
  spline S382 degree 2 poles (5.0405, 47.8412) (5.0405, 47.6455) (4.9603, 47.3306) (4.8764, 47.2139) knots 0 0 0 1 2 2 2
  spline S383 degree 2 poles (4.8764, 47.2139) (4.795, 47.0997) (4.5373, 46.972) (4.3683, 46.972) knots 0 0 0 1 2 2 2
  spline S384 degree 2 poles (4.3683, 46.972) (4.3185, 46.972) (4.231, 46.9818) (4.1981, 46.9927) knots 0 0 0 1 2 2 2
  line L494 (4.1981, 46.9927) -> (4.1981, 47.186)
  line L495 (4.1981, 47.186) -> (4.2066, 47.186)
  spline S385 degree 2 poles (4.2066, 47.186) (4.2346, 47.1714) (4.3367, 47.1459) (4.3951, 47.1459) knots 0 0 0 1 2 2 2
  spline S386 degree 2 poles (4.3951, 47.1459) (4.5823, 47.1459) (4.812, 47.3987) (4.8339, 47.6467) knots 0 0 0 1 2 2 2
  spline S387 degree 2 poles (4.8339, 47.6467) (4.7622, 47.5968) (4.6114, 47.5421) (4.5215, 47.5421) knots 0 0 0 1 2 2 2
  spline S388 degree 2 poles (4.5215, 47.5421) (4.434, 47.5421) (4.3027, 47.5774) (4.231, 47.6309) knots 0 0 0 1 2 2 2
  spline S389 degree 2 poles (4.231, 47.6309) (4.1483, 47.6929) (4.0681, 47.8849) (4.0681, 48.0138) knots 0 0 0 1 2 2 2
  spline S390 degree 2 poles (4.2723, 48.0223) (4.2723, 47.9299) (4.3209, 47.8047) (4.3744, 47.7609) knots 0 0 0 1 2 2 2
  spline S391 degree 2 poles (4.3744, 47.7609) (4.4145, 47.7293) (4.5142, 47.7087) (4.5665, 47.7087) knots 0 0 0 1 2 2 2
  spline S392 degree 2 poles (4.5665, 47.7087) (4.637, 47.7087) (4.7694, 47.7512) (4.8339, 47.7913) knots 0 0 0 1 2 2 2
  spline S393 degree 2 poles (4.8339, 47.7913) (4.8351, 47.8132) (4.8375, 47.8545) (4.8375, 47.8861) knots 0 0 0 1 2 2 2
  spline S394 degree 2 poles (4.8375, 47.8861) (4.8375, 48.0417) (4.7767, 48.2326) (4.7306, 48.2824) knots 0 0 0 1 2 2 2
  spline S395 degree 2 poles (4.7306, 48.2824) (4.688, 48.3298) (4.5956, 48.3675) (4.5434, 48.3675) knots 0 0 0 1 2 2 2
  spline S396 degree 2 poles (4.5434, 48.3675) (4.4218, 48.3675) (4.2723, 48.1949) (4.2723, 48.0223) knots 0 0 0 1 2 2 2
  spline S397 degree 2 poles (5.2605, 50.0677) (5.263, 50.1698) (5.3006, 50.3606) (5.342, 50.436) knots 0 0 0 1 2 2 2
  spline S398 degree 2 poles (5.342, 50.436) (5.3833, 50.5089) (5.5061, 50.6013) (5.6045, 50.6013) knots 0 0 0 1 2 2 2
  spline S399 degree 2 poles (5.6045, 50.6013) (5.6629, 50.6013) (5.7541, 50.5697) (5.7893, 50.5454) knots 0 0 0 1 2 2 2
  spline S400 degree 2 poles (5.7893, 50.5454) (5.8246, 50.5199) (5.889, 50.4494) (5.9145, 50.419) knots 0 0 0 1 2 2 2
  spline S401 degree 2 poles (5.9145, 50.419) (5.9412, 50.3861) (5.9935, 50.3169) (6.019, 50.2913) knots 0 0 0 1 2 2 2
  spline S402 degree 2 poles (6.019, 50.2913) (6.047, 50.2634) (6.1053, 50.2293) (6.1418, 50.2293) knots 0 0 0 1 2 2 2
  spline S403 degree 2 poles (6.1418, 50.2293) (6.1929, 50.2293) (6.2597, 50.2828) (6.2816, 50.3351) knots 0 0 0 1 2 2 2
  spline S404 degree 2 poles (6.2816, 50.3351) (6.3023, 50.3849) (6.3205, 50.5247) (6.3229, 50.6013) knots 0 0 0 1 2 2 2
  line L496 (6.3229, 50.6013) -> (6.4919, 50.6013)
  spline S405 degree 2 poles (6.4919, 50.6013) (6.4895, 50.4968) (6.4506, 50.3059) (6.4117, 50.233) knots 0 0 0 1 2 2 2
  spline S406 degree 2 poles (6.4117, 50.233) (6.3716, 50.1576) (6.2378, 50.0677) (6.1467, 50.0677) knots 0 0 0 1 2 2 2
  spline S407 degree 2 poles (6.1467, 50.0677) (6.0871, 50.0677) (5.9947, 50.0993) (5.9595, 50.1248) knots 0 0 0 1 2 2 2
  spline S408 degree 2 poles (5.9595, 50.1248) (5.9242, 50.1503) (5.8647, 50.2147) (5.8367, 50.25) knots 0 0 0 1 2 2 2
  spline S409 degree 2 poles (5.8367, 50.25) (5.8148, 50.2767) (5.7528, 50.3558) (5.7322, 50.3776) knots 0 0 0 1 2 2 2
  spline S410 degree 2 poles (5.7322, 50.3776) (5.703, 50.408) (5.6434, 50.4396) (5.6106, 50.4396) knots 0 0 0 1 2 2 2
  spline S411 degree 2 poles (5.6106, 50.4396) (5.5596, 50.4396) (5.4903, 50.3837) (5.4708, 50.3351) knots 0 0 0 1 2 2 2
  spline S412 degree 2 poles (5.4708, 50.3351) (5.4502, 50.2853) (5.4319, 50.1503) (5.4295, 50.0677) knots 0 0 0 1 2 2 2
  line L497 (5.4295, 50.0677) -> (5.2605, 50.0677)
  spline S413 degree 2 poles (4.107, 50.5235) (4.107, 50.6317) (4.1763, 50.8165) (4.2395, 50.8845) knots 0 0 0 1 2 2 2
  spline S414 degree 2 poles (4.2395, 50.8845) (4.3027, 50.9526) (4.4911, 51.0316) (4.6078, 51.0316) knots 0 0 0 1 2 2 2
  spline S415 degree 2 poles (4.6078, 51.0316) (4.7147, 51.0316) (4.9238, 50.9842) (5.0004, 50.9465) knots 0 0 0 1 2 2 2
  line L498 (5.0004, 50.9465) -> (5.0004, 50.7338)
  line L499 (5.0004, 50.7338) -> (4.9858, 50.7338)
  spline S416 degree 2 poles (4.9858, 50.7338) (4.9627, 50.7508) (4.8764, 50.7946) (4.8241, 50.814) knots 0 0 0 1 2 2 2
  spline S417 degree 2 poles (4.8241, 50.814) (4.7646, 50.8347) (4.6661, 50.8578) (4.6041, 50.8578) knots 0 0 0 1 2 2 2
  spline S418 degree 2 poles (4.6041, 50.8578) (4.5434, 50.8578) (4.4291, 50.814) (4.3878, 50.7666) knots 0 0 0 1 2 2 2
  spline S419 degree 2 poles (4.3878, 50.7666) (4.3501, 50.7216) (4.3112, 50.6025) (4.3112, 50.5223) knots 0 0 0 1 2 2 2
  spline S420 degree 2 poles (4.3112, 50.5223) (4.3112, 50.4421) (4.3549, 50.34) (4.3963, 50.3059) knots 0 0 0 1 2 2 2
  spline S421 degree 2 poles (4.3963, 50.3059) (4.4388, 50.2682) (4.5652, 50.2366) (4.6418, 50.2366) knots 0 0 0 1 2 2 2
  spline S422 degree 2 poles (4.6418, 50.2366) (4.7245, 50.2366) (4.8886, 50.2622) (4.9384, 50.2731) knots 0 0 0 1 2 2 2
  line L500 (4.9384, 50.2731) -> (4.9384, 49.5)
  line L501 (4.9384, 49.5) -> (4.1155, 49.5)
  line L502 (4.1155, 49.5) -> (4.1155, 49.6763)
  line L503 (4.1155, 49.6763) -> (4.7451, 49.6763)
  line L504 (4.7451, 49.6763) -> (4.7451, 50.0762)
  spline S423 degree 2 poles (4.7451, 50.0762) (4.7087, 50.0713) (4.6382, 50.0677) (4.609, 50.0677) knots 0 0 0 1 2 2 2
  spline S424 degree 2 poles (4.609, 50.0677) (4.4935, 50.0677) (4.3343, 50.1053) (4.2613, 50.1613) knots 0 0 0 1 2 2 2
  spline S425 degree 2 poles (4.2613, 50.1613) (4.1872, 50.2172) (4.107, 50.3874) (4.107, 50.5235) knots 0 0 0 1 2 2 2
  line L505 (4.0511, 52.9846) -> (4.2297, 52.9846)
  line L506 (4.2297, 52.9846) -> (4.2297, 53.5)
  line L507 (4.2297, 53.5) -> (4.423, 53.5)
  line L508 (4.423, 53.5) -> (4.423, 52.9846)
  line L509 (4.423, 52.9846) -> (5.0855, 52.9846)
  line L510 (5.0855, 52.9846) -> (5.0855, 52.7731)
  line L511 (5.0855, 52.7731) -> (4.4145, 52)
  line L512 (4.4145, 52) -> (4.2297, 52)
  line L513 (4.2297, 52) -> (4.2297, 52.8229)
  line L514 (4.2297, 52.8229) -> (4.0511, 52.8229)
  line L515 (4.0511, 52.8229) -> (4.0511, 52.9846)
  line L516 (4.423, 52.8229) -> (4.423, 52.237)
  line L517 (4.423, 52.237) -> (4.9275, 52.8229)
  line L518 (4.9275, 52.8229) -> (4.423, 52.8229)
  spline S426 degree 2 poles (5.2605, 55.0677) (5.263, 55.1698) (5.3006, 55.3606) (5.342, 55.436) knots 0 0 0 1 2 2 2
  spline S427 degree 2 poles (5.342, 55.436) (5.3833, 55.5089) (5.5061, 55.6013) (5.6045, 55.6013) knots 0 0 0 1 2 2 2
  spline S428 degree 2 poles (5.6045, 55.6013) (5.6629, 55.6013) (5.7541, 55.5697) (5.7893, 55.5454) knots 0 0 0 1 2 2 2
  spline S429 degree 2 poles (5.7893, 55.5454) (5.8246, 55.5199) (5.889, 55.4494) (5.9145, 55.419) knots 0 0 0 1 2 2 2
  spline S430 degree 2 poles (5.9145, 55.419) (5.9412, 55.3861) (5.9935, 55.3169) (6.019, 55.2913) knots 0 0 0 1 2 2 2
  spline S431 degree 2 poles (6.019, 55.2913) (6.047, 55.2634) (6.1053, 55.2293) (6.1418, 55.2293) knots 0 0 0 1 2 2 2
  spline S432 degree 2 poles (6.1418, 55.2293) (6.1929, 55.2293) (6.2597, 55.2828) (6.2816, 55.3351) knots 0 0 0 1 2 2 2
  spline S433 degree 2 poles (6.2816, 55.3351) (6.3023, 55.3849) (6.3205, 55.5247) (6.3229, 55.6013) knots 0 0 0 1 2 2 2
  line L519 (6.3229, 55.6013) -> (6.4919, 55.6013)
  spline S434 degree 2 poles (6.4919, 55.6013) (6.4895, 55.4968) (6.4506, 55.3059) (6.4117, 55.233) knots 0 0 0 1 2 2 2
  spline S435 degree 2 poles (6.4117, 55.233) (6.3716, 55.1576) (6.2378, 55.0677) (6.1467, 55.0677) knots 0 0 0 1 2 2 2
  spline S436 degree 2 poles (6.1467, 55.0677) (6.0871, 55.0677) (5.9947, 55.0993) (5.9595, 55.1248) knots 0 0 0 1 2 2 2
  spline S437 degree 2 poles (5.9595, 55.1248) (5.9242, 55.1503) (5.8647, 55.2147) (5.8367, 55.25) knots 0 0 0 1 2 2 2
  spline S438 degree 2 poles (5.8367, 55.25) (5.8148, 55.2767) (5.7528, 55.3558) (5.7322, 55.3776) knots 0 0 0 1 2 2 2
  spline S439 degree 2 poles (5.7322, 55.3776) (5.703, 55.408) (5.6434, 55.4396) (5.6106, 55.4396) knots 0 0 0 1 2 2 2
  spline S440 degree 2 poles (5.6106, 55.4396) (5.5596, 55.4396) (5.4903, 55.3837) (5.4708, 55.3351) knots 0 0 0 1 2 2 2
  spline S441 degree 2 poles (5.4708, 55.3351) (5.4502, 55.2853) (5.4319, 55.1503) (5.4295, 55.0677) knots 0 0 0 1 2 2 2
  line L520 (5.4295, 55.0677) -> (5.2605, 55.0677)
  spline S442 degree 2 poles (4.6114, 54.6422) (4.6661, 54.6422) (4.7743, 54.669) (4.8266, 54.6896) knots 0 0 0 1 2 2 2
  spline S443 degree 2 poles (4.8266, 54.6896) (4.8752, 54.7103) (4.9469, 54.7541) (4.9749, 54.7735) knots 0 0 0 1 2 2 2
  line L521 (4.9749, 54.7735) -> (4.987, 54.7735)
  line L522 (4.987, 54.7735) -> (4.987, 54.5608)
  spline S444 degree 2 poles (4.987, 54.5608) (4.9214, 54.5255) (4.6965, 54.4684) (4.5956, 54.4684) knots 0 0 0 1 2 2 2
  spline S445 degree 2 poles (4.5956, 54.4684) (4.4935, 54.4684) (4.3416, 54.5097) (4.2796, 54.5535) knots 0 0 0 1 2 2 2
  spline S446 degree 2 poles (4.2796, 54.5535) (4.2139, 54.6009) (4.1459, 54.7382) (4.1459, 54.8306) knots 0 0 0 1 2 2 2
  spline S447 degree 2 poles (4.1459, 54.8306) (4.1459, 54.9546) (4.3088, 55.1418) (4.423, 55.1661) knots 0 0 0 1 2 2 2
  line L523 (4.423, 55.1661) -> (4.423, 55.1807)
  spline S448 degree 2 poles (4.423, 55.1807) (4.3756, 55.1904) (4.2674, 55.2342) (4.2212, 55.278) knots 0 0 0 1 2 2 2
  spline S449 degree 2 poles (4.2212, 55.278) (4.175, 55.3205) (4.1167, 55.4566) (4.1167, 55.5551) knots 0 0 0 1 2 2 2
  spline S450 degree 2 poles (4.1167, 55.5551) (4.1167, 55.656) (4.186, 55.8274) (4.2492, 55.893) knots 0 0 0 1 2 2 2
  spline S451 degree 2 poles (4.2492, 55.893) (4.3148, 55.9611) (4.5008, 56.0316) (4.6187, 56.0316) knots 0 0 0 1 2 2 2
  spline S452 degree 2 poles (4.6187, 56.0316) (4.7318, 56.0316) (4.953, 55.9769) (5.0284, 55.9392) knots 0 0 0 1 2 2 2
  line L524 (5.0284, 55.9392) -> (5.0284, 55.7265)
  line L525 (5.0284, 55.7265) -> (5.0138, 55.7265)
  spline S453 degree 2 poles (5.0138, 55.7265) (4.9506, 55.7727) (4.7366, 55.8578) (4.6309, 55.8578) knots 0 0 0 1 2 2 2
  spline S454 degree 2 poles (4.6309, 55.8578) (4.5689, 55.8578) (4.4449, 55.8189) (4.4036, 55.7739) knots 0 0 0 1 2 2 2
  spline S455 degree 2 poles (4.4036, 55.7739) (4.3635, 55.7289) (4.3209, 55.622) (4.3209, 55.5405) knots 0 0 0 1 2 2 2
  spline S456 degree 2 poles (4.3209, 55.5405) (4.3209, 55.4591) (4.3683, 55.3533) (4.4109, 55.3229) knots 0 0 0 1 2 2 2
  spline S457 degree 2 poles (4.4109, 55.3229) (4.4534, 55.2925) (4.5689, 55.2694) (4.637, 55.2694) knots 0 0 0 1 2 2 2
  line L526 (4.637, 55.2694) -> (4.722, 55.2694)
  line L527 (4.722, 55.2694) -> (4.722, 55.1029)
  line L528 (4.722, 55.1029) -> (4.6552, 55.1029)
  spline S458 degree 2 poles (4.6552, 55.1029) (4.5203, 55.1029) (4.3501, 54.9741) (4.3501, 54.8513) knots 0 0 0 1 2 2 2
  spline S459 degree 2 poles (4.3501, 54.8513) (4.3501, 54.7942) (4.3938, 54.7127) (4.4291, 54.6884) knots 0 0 0 1 2 2 2
  spline S460 degree 2 poles (4.4291, 54.6884) (4.4668, 54.6629) (4.5592, 54.6422) (4.6114, 54.6422) knots 0 0 0 1 2 2 2
  line L529 (4.0912, 58.5) -> (5.0162, 58.5)
  line L530 (5.0162, 58.5) -> (5.0162, 58.2873)
  spline S461 degree 2 poles (5.0162, 58.2873) (4.9165, 58.1937) (4.7391, 58.0199) (4.654, 57.9263) knots 0 0 0 1 2 2 2
  spline S462 degree 2 poles (4.654, 57.9263) (4.4826, 57.7378) (4.3574, 57.5118) (4.3574, 57.3914) knots 0 0 0 1 2 2 2
  spline S463 degree 2 poles (4.3574, 57.3914) (4.3574, 57.3282) (4.3963, 57.2334) (4.4315, 57.203) knots 0 0 0 1 2 2 2
  spline S464 degree 2 poles (4.4315, 57.203) (4.4668, 57.1726) (4.5592, 57.1422) (4.6151, 57.1422) knots 0 0 0 1 2 2 2
  spline S465 degree 2 poles (4.6151, 57.1422) (4.6686, 57.1422) (4.778, 57.169) (4.8278, 57.1896) knots 0 0 0 1 2 2 2
  spline S466 degree 2 poles (4.8278, 57.1896) (4.8703, 57.2066) (4.9494, 57.2553) (4.9737, 57.2723) knots 0 0 0 1 2 2 2
  line L531 (4.9737, 57.2723) -> (4.9846, 57.2723)
  line L532 (4.9846, 57.2723) -> (4.9846, 57.0583)
  spline S467 degree 2 poles (4.9846, 57.0583) (4.9226, 57.028) (4.7002, 56.9684) (4.6005, 56.9684) knots 0 0 0 1 2 2 2
  spline S468 degree 2 poles (4.6005, 56.9684) (4.3902, 56.9684) (4.1532, 57.1908) (4.1532, 57.3805) knots 0 0 0 1 2 2 2
  spline S469 degree 2 poles (4.1532, 57.3805) (4.1532, 57.4692) (4.1945, 57.6175) (4.231, 57.6807) knots 0 0 0 1 2 2 2
  spline S470 degree 2 poles (4.231, 57.6807) (4.2674, 57.7464) (4.3732, 57.8752) (4.4315, 57.9372) knots 0 0 0 1 2 2 2
  spline S471 degree 2 poles (4.4315, 57.9372) (4.5263, 58.0405) (4.7585, 58.2618) (4.8278, 58.3262) knots 0 0 0 1 2 2 2
  line L533 (4.8278, 58.3262) -> (4.0912, 58.3262)
  line L534 (4.0912, 58.3262) -> (4.0912, 58.5)
  line L535 (8.5401, 61) -> (8.799, 61)
  line L536 (8.799, 61) -> (9.2731, 60.4032)
  line L537 (9.2731, 60.4032) -> (9.5016, 60.4032)
  line L538 (9.5016, 60.4032) -> (9.5016, 61)
  line L539 (9.5016, 61) -> (9.701, 61)
  line L540 (9.701, 61) -> (9.701, 59.5)
  line L541 (9.701, 59.5) -> (9.3144, 59.5)
  spline S472 degree 2 poles (9.3144, 59.5) (9.1856, 59.5) (9.0118, 59.528) (8.9327, 59.579) knots 0 0 0 1 2 2 2
  spline S473 degree 2 poles (8.9327, 59.579) (8.8537, 59.6301) (8.7626, 59.7893) (8.7626, 59.9072) knots 0 0 0 1 2 2 2
  spline S474 degree 2 poles (8.7626, 59.9072) (8.7626, 60.0713) (8.9303, 60.2938) (9.0737, 60.3472) knots 0 0 0 1 2 2 2
  line L542 (9.0737, 60.3472) -> (8.5401, 61)
  spline S475 degree 2 poles (8.9704, 59.923) (8.9704, 59.8574) (9.0166, 59.7565) (9.0652, 59.7237) knots 0 0 0 1 2 2 2
  spline S476 degree 2 poles (9.0652, 59.7237) (9.1078, 59.6957) (9.2208, 59.6726) (9.3035, 59.6726) knots 0 0 0 1 2 2 2
  line L543 (9.3035, 59.6726) -> (9.5016, 59.6726)
  line L544 (9.5016, 59.6726) -> (9.5016, 60.2366)
  line L545 (9.5016, 60.2366) -> (9.3266, 60.2366)